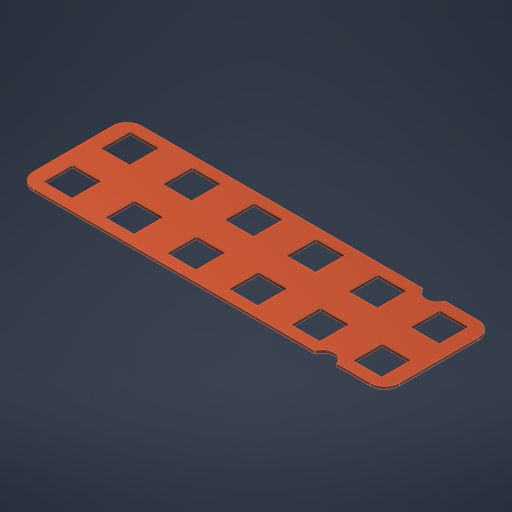
# Autodesk Inventor part: bat_contacts_v2_plate
Saved by Autodesk Inventor 2024.3 (Build 283343010, 343A)
## iProperties
Created: 2025-05-07
Part Number: bat_contacts_v2_plate
Material: Kupfer
Document SubType Name: Modellieren
Designer: David
Density: 8.94 g/cm^3
Appearance: Kupfer - satiniert
Sheet Metal Rule: Standard_mm
Author: David
Autodesk Inventor part; units mm, degrees
ref_plane "YZ Plane" through (0, 0, 0) normal (1, 0, 0) x (0, 1, 0)
ref_plane "XZ Plane" through (0, 0, 0) normal (0, 1, 0) x (-1, 0, 0)
ref_plane "XY Plane" through (0, 0, 0) normal (0, 0, 1) x (1, 0, 0)
sketch "Skizze1" plane through (0, 0, 0) normal (0, 0, 1) x (1, 0, 0)
  line L0 (0, 0) -> (127, 0)
  line L1 (127, 0) -> (127, 37.5)
  line L2 (127, 37.5) -> (0, 37.5)
  line L3 (0, 37.5) -> (0, 0)
  line L4 (4.75, 3.65) -> (14.75, 3.65)
  line L5 (14.75, 3.65) -> (14.75, 13.85)
  line L6 (14.75, 13.85) -> (4.75, 13.85)
  line L7 (4.75, 13.85) -> (4.75, 3.65)
  line L8 (4.75, 33.85) -> (4.75, 23.65)
  line L9 (14.75, 33.85) -> (4.75, 33.85)
  line L10 (14.75, 23.65) -> (14.75, 33.85)
  line L11 (4.75, 23.65) -> (14.75, 23.65)
  line L12 (26.25, 13.85) -> (26.25, 3.65)
  line L13 (36.25, 13.85) -> (26.25, 13.85)
  line L14 (36.25, 3.65) -> (36.25, 13.85)
  line L15 (26.25, 3.65) -> (36.25, 3.65)
  line L16 (26.25, 33.85) -> (26.25, 23.65)
  line L17 (36.25, 33.85) -> (26.25, 33.85)
  line L18 (36.25, 23.65) -> (36.25, 33.85)
  line L19 (26.25, 23.65) -> (36.25, 23.65)
  line L20 (47.75, 13.85) -> (47.75, 3.65)
  line L21 (57.75, 13.85) -> (47.75, 13.85)
  line L22 (57.75, 3.65) -> (57.75, 13.85)
  line L23 (47.75, 3.65) -> (57.75, 3.65)
  line L24 (47.75, 33.85) -> (47.75, 23.65)
  line L25 (57.75, 33.85) -> (47.75, 33.85)
  line L26 (57.75, 23.65) -> (57.75, 33.85)
  line L27 (47.75, 23.65) -> (57.75, 23.65)
  line L28 (69.25, 13.85) -> (69.25, 3.65)
  line L29 (79.25, 13.85) -> (69.25, 13.85)
  line L30 (79.25, 3.65) -> (79.25, 13.85)
  line L31 (69.25, 3.65) -> (79.25, 3.65)
  line L32 (69.25, 33.85) -> (69.25, 23.65)
  line L33 (79.25, 33.85) -> (69.25, 33.85)
  line L34 (79.25, 23.65) -> (79.25, 33.85)
  line L35 (69.25, 23.65) -> (79.25, 23.65)
  line L36 (90.75, 13.85) -> (90.75, 3.65)
  line L37 (100.75, 13.85) -> (90.75, 13.85)
  line L38 (100.75, 3.65) -> (100.75, 13.85)
  line L39 (90.75, 3.65) -> (100.75, 3.65)
  line L40 (90.75, 33.85) -> (90.75, 23.65)
  line L41 (100.75, 33.85) -> (90.75, 33.85)
  line L42 (100.75, 23.65) -> (100.75, 33.85)
  line L43 (90.75, 23.65) -> (100.75, 23.65)
  line L44 (112.25, 13.85) -> (112.25, 3.65)
  line L45 (122.25, 13.85) -> (112.25, 13.85)
  line L46 (122.25, 3.65) -> (122.25, 13.85)
  line L47 (112.25, 3.65) -> (122.25, 3.65)
  line L48 (112.25, 33.85) -> (112.25, 23.65)
  line L49 (122.25, 33.85) -> (112.25, 33.85)
  line L50 (122.25, 23.65) -> (122.25, 33.85)
  line L51 (112.25, 23.65) -> (122.25, 23.65)
  arc A0 (110.2997, 0) -> (102.7003, 0) centre (106.5, -1.25) ccw
  arc A1 (102.7003, 37.5) -> (110.2997, 37.5) centre (106.5, 38.75) ccw
  point P0 (0, 18.75)
  point P1 (63.5, 37.5)
  point P2 (42, 18.75)
  point P3 (85, 18.75)
  point P4 (63.5, 0)
  point P5 (4.75, 28.75)
  point P6 (95.75, 3.65)
  dimension "d0" = 127
  dimension "d1" = 37.5
  dimension "d2" = 10.2
  dimension "d3" = 10
  dimension "d6" = 20
  dimension "d9" = 21.5
  dimension "d13" = 5.75
  dimension "d17" = 43
  dimension "d18" = 21.5
  dimension "d19" = 10
  dimension "d20" = 4
  dimension "d21" = 1.25
  dimension "d22" = 10.75
  dimension "d23" = 1.25
  constraints: 104 end point, 5 midpoint, 4 parallel, 4 point on circle, 4 point on line, 3 horizontal, 2 centre point, 2 horizontal alignment, 2 perpendicular, 1 equal radius, 1 vertical, 1 vertical alignment, 88 other
  measures "d0" distance of L1.end L2.end
  measures "d1" distance of L2.end L0.start
  measures "d2" distance of L6.end L4.start
  measures "d3" distance of L4.start L4.end
  measures "d6" distance of L6.end L8.start
  measures "d9" distance of L6.end L12.start
  measures "d13" distance from line of point (63.5, 37.5) L26
  measures "d17" distance of point (85, 18.75) point (42, 18.75)
  measures "d18" horizontal distance of point (63.5, 0) point (42, 18.75)
  measures "d19" vertical distance of point (0, 18.75) point (4.75, 28.75)
  measures "d20" radius of A0
  measures "d21" distance from line of L0 A0.centre
  measures "d22" horizontal distance of point (95.75, 3.65) A0.centre
  measures "d23" distance from line of L2 A1.centre
extrude "Extrusion1" add sketch "Skizze1" along normal blind 1 contours L3 L2 A1 L1 L0 A0
fillet "Rundung1" radius 5 4 edges at (127, 37.5, 0.5) (127, 0, 0.5) (0, 37.5, 0.5) (0, 0, 0.5)
sketch "Skizze2" plane through (0, 0, 1) normal (0, 0, 1) x (1, 0, 0)
  arc A0 (0, 5) -> (5, 0) centre (5, 5) ccw projected
  line L0 (5, 0) -> (102.7003, 0) projected
  arc A1 (122, 0) -> (127, 5) centre (122, 5) ccw projected
  line L1 (127, 5) -> (127, 32.5) projected
  arc A2 (127, 32.5) -> (122, 37.5) centre (122, 32.5) ccw projected
  line L2 (122, 37.5) -> (110.2997, 37.5) projected
  arc A3 (5, 37.5) -> (0, 32.5) centre (5, 32.5) ccw projected
  line L3 (0, 32.5) -> (0, 5) projected
  line L4 (112.25, 33.85) -> (122.25, 33.85) projected
  line L5 (122.25, 33.85) -> (122.25, 23.65) projected
  line L6 (122.25, 23.65) -> (112.25, 23.65) projected
  line L7 (112.25, 23.65) -> (112.25, 33.85) projected
  line L8 (112.25, 13.85) -> (122.25, 13.85) projected
  line L9 (122.25, 13.85) -> (122.25, 3.65) projected
  line L10 (122.25, 3.65) -> (112.25, 3.65) projected
  line L11 (112.25, 3.65) -> (112.25, 13.85) projected
  line L12 (90.75, 33.85) -> (100.75, 33.85) projected
  line L13 (100.75, 33.85) -> (100.75, 23.65) projected
  line L14 (100.75, 23.65) -> (90.75, 23.65) projected
  line L15 (90.75, 23.65) -> (90.75, 33.85) projected
  line L16 (90.75, 13.85) -> (100.75, 13.85) projected
  line L17 (100.75, 13.85) -> (100.75, 3.65) projected
  line L18 (100.75, 3.65) -> (90.75, 3.65) projected
  line L19 (90.75, 3.65) -> (90.75, 13.85) projected
  line L20 (69.25, 33.85) -> (79.25, 33.85) projected
  line L21 (79.25, 33.85) -> (79.25, 23.65) projected
  line L22 (79.25, 23.65) -> (69.25, 23.65) projected
  line L23 (69.25, 23.65) -> (69.25, 33.85) projected
  line L24 (69.25, 13.85) -> (79.25, 13.85) projected
  line L25 (79.25, 13.85) -> (79.25, 3.65) projected
  line L26 (79.25, 3.65) -> (69.25, 3.65) projected
  line L27 (69.25, 3.65) -> (69.25, 13.85) projected
  line L28 (47.75, 33.85) -> (57.75, 33.85) projected
  line L29 (57.75, 33.85) -> (57.75, 23.65) projected
  line L30 (57.75, 23.65) -> (47.75, 23.65) projected
  line L31 (47.75, 23.65) -> (47.75, 33.85) projected
  line L32 (47.75, 13.85) -> (57.75, 13.85) projected
  line L33 (57.75, 13.85) -> (57.75, 3.65) projected
  line L34 (57.75, 3.65) -> (47.75, 3.65) projected
  line L35 (47.75, 3.65) -> (47.75, 13.85) projected
  line L36 (26.25, 33.85) -> (36.25, 33.85) projected
  line L37 (36.25, 33.85) -> (36.25, 23.65) projected
  line L38 (36.25, 23.65) -> (26.25, 23.65) projected
  line L39 (26.25, 23.65) -> (26.25, 33.85) projected
  line L40 (26.25, 13.85) -> (36.25, 13.85) projected
  line L41 (36.25, 13.85) -> (36.25, 3.65) projected
  line L42 (36.25, 3.65) -> (26.25, 3.65) projected
  line L43 (26.25, 3.65) -> (26.25, 13.85) projected
  line L44 (4.75, 33.85) -> (14.75, 33.85) projected
  line L45 (14.75, 33.85) -> (14.75, 23.65) projected
  line L46 (14.75, 23.65) -> (4.75, 23.65) projected
  line L47 (4.75, 23.65) -> (4.75, 33.85) projected
  line L48 (4.75, 3.65) -> (4.75, 13.85) projected
  line L49 (4.75, 13.85) -> (14.75, 13.85) projected
  line L50 (14.75, 13.85) -> (14.75, 3.65) projected
  line L51 (14.75, 3.65) -> (4.75, 3.65) projected
  arc A4 (110.2997, 0) -> (102.7003, 0) centre (106.5, -1.25) ccw projected
  line L52 (110.2997, 0) -> (122, 0) projected
  arc A5 (102.7003, 37.5) -> (110.2997, 37.5) centre (106.5, 38.75) ccw projected
  line L53 (102.7003, 37.5) -> (5, 37.5) projected
  point P0 (0, 0)
equation "\"d13\" = -0.5 * d3 + 0.5 * d9"
equation "\"d17\" = 2 * d9"
equation "\"d18\" = 0.5 * d17"
equation "\"d19\" = 0.5 * d6"
equation "\"d22\" = 0.5 * d18"
equation "\"d23\" = d21"
equation "\"Biegeradius\" = Stärke"
equation "\"BreiteBiegungsfreistellung\" = Stärke"
equation "\"TiefeBiegungsfreistellung\" = 0.5 * Stärke"
equation "\"GrößeEckenfreistellung\" = 4 * Stärke"
equation "\"MinimalRest\" = 2 * Stärke"
equation "\"Übergangsradius\" = Biegeradius"
equation "\"JacobiRadiusGröße\" = Biegeradius"
equation "\"Abstandsgröße\" = Stärke"
equation "\"Stärke\" = 0.5"
